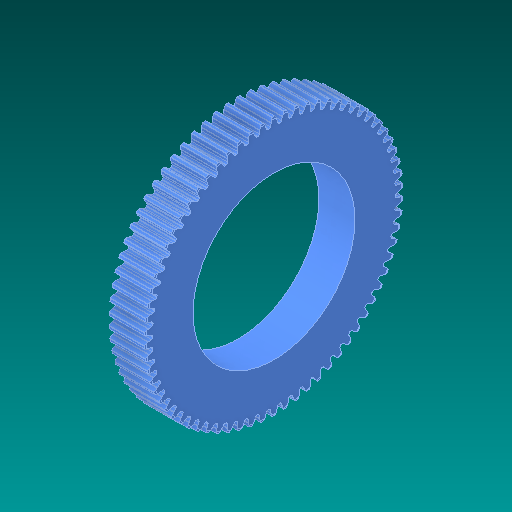
# Autodesk Inventor part: GEYK1.0-70-10-B-10K.0_t
Saved by Autodesk Inventor 2020 (Build 240168000, 168)
## iProperties
Created: 2022-11-14
Part Number: GEYK1.0-70-10-B-10K.0_t
Material: Generic
Catalog Web Link: www.cadenas.de
Description: GEY_teeth-Plastic Bonded Spur Gears
Vendor: MISUMI
Document SubType Name: Modeling
Designer: psAdmin
Manufacturer: MISUMI
Mass: 22.3714 g
Surface Area: 101.789 cm^2
Volume: 22.3714 cm^3
Density: 1 g/cm^3
Appearance: PSOLRGB-87-140-238
Category: PARTsolutions
Company: MISUMI
PSOL_IDENT_0: {$CADENAS_DATA/23d-libs/misumi/metric/54_spur_gears/gey_teeth.prj},214 {VTYP=3D},{NB=GEYK1.0-70-10-B
PSOL_IDENT_1: -10K.0_t},{LINA=GEYK1.0-70-10-B-10K.0},{NN=GEY_teeth},{DATE=07.06.2021 01:25:59},{GEOMDATE=22.08.201
PSOL_IDENT_2: 6 07:24:18},{VERSION=},{LINEID=10},{WBVAR=SHS,NT,PS,ALT1,ALT2,BS},{WBNUMERIC=NT,BS}  {NB=GEYK1.0-70-
PSOL_IDENT_3: 10-B-10K.0_t},{LINA=GEYK1.0-70-10-B-10K.0},{KT=DUMMY},{PN=GEYK1.0-70-10-B-10K.0},{SHS=K},{SHSPN=K},{
PSOL_IDENT_4: GEAKBH=0},{MAT=MC Nylon},{MATC=S25C},{AC=Set Screw},{MOD=1.0},{NT=70},{NTA=30,32,34,35,36,38,40,42,4
PSOL_IDENT_5: 5,48,50,52,56,60,70,75},{B=10},{TS=B},{TSA='B','B'},{PS=10K},{PSA= '10N','10N','10K','10K','11N','11
PSOL_IDENT_6: N','12N','12N','13N','13N','14N','14N','15N','15N','16N','16N','17N','17N','18N','18N','19N','19N','
PSOL_IDENT_7: 20N','20N','21N','21N','22N','22N','23N','23N','24N','24N'},{PS1= '10','10','11','11','12','12','13'
PSOL_IDENT_8: ,'13','14','14','15','15','16','16','17','17','18','18','19','19','20','20','21','21','22','22','23'
PSOL_IDENT_9: ,'23','24','24','25','25','26','26','27','27','28','28'},{PS2= '10N','10N','10K','10K','11N','11N','
PSOL_IDENT_10: 12N','12N','13N','13N','14N','14N','15N','15N','16N','16N','17N','17N','18N','18N','19N','19N','20N'
PSOL_IDENT_11: ,'20N','21N','21N','22N','22N','23N','23N','24N','24N'},{P=10.00},{DD=70.0},{D=72.0},{G=67.5},{H=40}
PSOL_IDENT_12: ,{E=45},{L=20},{LL1=10},{LL2=5.000},{M=M4},{M2=4},{ACSS=M4x3},{TT=0},{BB=4},{ALT1=},{ALTA='','w/o Se
PSOL_IDENT_13: t Screw', '-KC90', 'with KC90 (Set Screw)', '-KC120', 'with KC120 (Set Screw)'},{SCREWL=3},{PLANE=20
PSOL_IDENT_14: },{PLANE1=20},{ALT2=},{ALT2A='','w/o Boss Cut','-BS','with BS (Boss Cut)'},{BS=0.0},{BSA=0},{BSMIN=7
PSOL_IDENT_15: .0},{BSMAX=9.5},{MOD3D=1},{D1=1.285714},{D2=2.571429},{D3=20},{D4=0.1},{D5=11.666667},{D6=10.769231}
PSOL_IDENT_16: ,{D7=0.85},{D8=0.5},{D9=0.82917},{S1=15},{S2=0.5}
NB: GEYK1.0-70-10-B-10K.0_t
NN: GEY_teeth
NT: 70
NBSYN: $PN._t
LINA: GEYK1.0-70-10-B-10K.0
CATALOG: Misumi
SHS: Key Groove Hole+Tap
MAT: MC Nylon
MATC: S25C
MOD: 1.0
B: 10
PS: 10K
L: 20
LL1: 10
ALT1: w/o Set Screw
ALT2: w/o Boss Cut
BS: 0
SUPPLIER: MISUMI
ARTICLENO: GEYK1.0-70-10-B-10K.0_t
BOMINFO: GEYK1.0-70-10-B-10K.0
CREATOR: CADENAS GmbH
d3: 0.000 mm
Title: GEYK1.0-70-10-B-10K.0
Author: Cadenas PARTsolutions
Comments: Plastic Bonded Spur Gears
Autodesk Inventor part; units mm, degrees
(part 1 of 2)
sketch "_____2" plane through (0, 0, 0) normal (0, 0, 1) x (1, 0, 0)
  line L0 (0, 0) -> (-10, 0)
  line L1 (-10, 22.5) -> (0, 22.5)
  line L2 (0, 22.5) -> (0, 35.5)
  line L3 (0, 35.5) -> (-0.6699, 38)
  line L4 (-0.6699, 38) -> (-9.3301, 38)
  line L5 (-9.3301, 38) -> (-10, 35.5)
  line L6 (-10, 35.5) -> (-10, 22.5)
  constraints: 14 end point
revolve "Revolution1" add sketch "_____2" angle 360 about axis through (0, 0, 0) along (1, 0, 0)
sketch "Sketch_2" plane through (0, 0, 0) normal (1, 0, 0) x (0, 1, 0)
  circle A0 centre (0, 0) radius 144
  arc A1 (1.2884, 35.9769) -> (1.1952, 35.9213) centre (1.2849, 35.877) ccw
  arc A2 (1.1952, 35.9213) -> (0.7853, 34.9912) centre (11.6561, 30.756) ccw
  arc A3 (0.7853, 34.9912) -> (0.7497, 34.8755) centre (1.5579, 34.6902) ccw
  arc A4 (0.5416, 34.1021) -> (0.7497, 34.8755) centre (-9.7463, 37.2859) ccw
  arc A5 (0.063, 33.7499) -> (0.5416, 34.1021) centre (0.0639, 34.2499) ccw
  arc A6 (0.063, 33.7499) -> (-0.063, 33.7499) centre (0, 0) ccw
  arc A7 (-0.5416, 34.1021) -> (-0.063, 33.7499) centre (-0.0639, 34.2499) ccw
  arc A8 (-0.7497, 34.8755) -> (-0.5416, 34.1021) centre (9.7463, 37.2859) ccw
  arc A9 (-0.7497, 34.8755) -> (-0.7853, 34.9912) centre (-1.5579, 34.6902) ccw
  arc A10 (-0.7853, 34.9912) -> (-1.1952, 35.9213) centre (-11.6561, 30.756) ccw
  arc A11 (-1.1952, 35.9213) -> (-1.2884, 35.9769) centre (-1.2849, 35.877) ccw
  arc A12 (-1.2884, 35.9769) -> (-1.9417, 35.9476) centre (0, 0) ccw
  arc A13 (-1.9417, 35.9476) -> (-2.0296, 35.8838) centre (-1.9363, 35.8477) ccw
  arc A14 (-2.0296, 35.8838) -> (-2.3544, 34.9207) centre (8.8523, 31.677) ccw
  arc A15 (-2.3544, 34.9207) -> (-2.3795, 34.8023) centre (-1.5579, 34.6902) ccw
  arc A16 (-2.5175, 34.0134) -> (-2.3795, 34.8023) centre (-13.0493, 36.2622) ccw
  arc A17 (-2.9626, 33.6197) -> (-2.5175, 34.0134) centre (-3.0065, 34.1178) ccw
  arc A18 (-2.9626, 33.6197) -> (-3.0881, 33.6084) centre (0, 0) ccw
  arc A19 (-3.5963, 33.9163) -> (-3.0881, 33.6084) centre (-3.1338, 34.1063) ccw
  arc A20 (-3.8729, 34.6679) -> (-3.5963, 33.9163) centre (6.3647, 38.0095) ccw
  arc A21 (-3.8729, 34.6679) -> (-3.9188, 34.7799) centre (-4.6613, 34.4109) ccw
  arc A22 (-3.9188, 34.7799) -> (-4.4104, 35.6695) centre (-14.3661, 29.5873) ccw
  arc A23 (-4.4104, 35.6695) -> (-4.5082, 35.7166) centre (-4.4957, 35.6174) ccw
  arc A24 (-4.5082, 35.7166) -> (-5.1562, 35.6288) centre (0, 0) ccw
  arc A25 (-5.1562, 35.6288) -> (-5.238, 35.5574) centre (-5.1419, 35.5299) ccw
  arc A26 (-5.238, 35.5574) -> (-5.4752, 34.5691) centre (5.9771, 32.343) ccw
  arc A27 (-5.4752, 34.5691) -> (-5.4896, 34.4489) centre (-4.6613, 34.4109) ccw
  arc A28 (-5.5563, 33.6508) -> (-5.4896, 34.4489) centre (-16.2473, 34.9465) ccw
  arc A29 (-5.9643, 33.2188) -> (-5.5563, 33.6508) centre (-6.0527, 33.7109) ccw
  arc A30 (-5.9643, 33.2188) -> (-6.0883, 33.1963) centre (0, 0) ccw
  arc A31 (-6.622, 33.4574) -> (-6.0883, 33.1963) centre (-6.1785, 33.6881) ccw
  arc A32 (-6.965, 34.1812) -> (-6.622, 33.4574) centre (2.932, 38.427) ccw
  arc A33 (-6.965, 34.1812) -> (-7.0206, 34.2886) centre (-7.7271, 33.8545) ccw
  arc A34 (-7.0206, 34.2886) -> (-7.59, 35.1306) centre (-16.9605, 28.1804) ccw
  arc A35 (-7.59, 35.1306) -> (-7.6917, 35.1687) centre (-7.6703, 35.071) ccw
  arc A36 (-7.6917, 35.1687) -> (-8.3292, 35.0232) centre (0, 0) ccw
  arc A37 (-8.3292, 35.0232) -> (-8.4042, 34.9447) centre (-8.306, 34.9259) ccw
  arc A38 (-8.4042, 34.9447) -> (-8.5519, 33.9391) centre (3.0538, 32.7486) ccw
  arc A39 (-8.5519, 33.9391) -> (-8.5554, 33.8182) centre (-7.7271, 33.8545) ccw
  arc A40 (-8.5504, 33.0173) -> (-8.5554, 33.8182) centre (-19.3145, 33.3494) ccw
  arc A41 (-8.918, 32.5504) -> (-8.5504, 33.0173) centre (-9.0501, 33.0327) ccw
  arc A42 (-8.918, 32.5504) -> (-9.0395, 32.5169) centre (0, 0) ccw
  arc A43 (-9.5945, 32.7291) -> (-9.0395, 32.5169) centre (-9.1734, 32.9987) ccw
  arc A44 (-10.0009, 33.4192) -> (-9.5945, 32.7291) centre (-0.5244, 38.5351) ccw
  arc A45 (-10.0009, 33.4192) -> (-10.066, 33.5213) centre (-10.7307, 33.0256) ccw
  arc A46 (-10.066, 33.5213) -> (-10.7085, 34.3088) centre (-19.4183, 26.5467) ccw
  arc A47 (-10.7085, 34.3088) -> (-10.8132, 34.3377) centre (-10.7832, 34.2423) ccw
  arc A48 (-10.8132, 34.3377) -> (-11.4351, 34.1356) centre (0, 0) ccw
  arc A49 (-11.4351, 34.1356) -> (-11.5028, 34.0507) centre (-11.4033, 34.0408) ccw
  arc A50 (-11.5028, 34.0507) -> (-11.5598, 33.0359) centre (0.106, 32.8905) ccw
  arc A51 (-11.5598, 33.0359) -> (-11.5524, 32.9151) centre (-10.7307, 33.0256) ccw
  arc A52 (-11.4756, 32.1179) -> (-11.5524, 32.9151) centre (-22.2261, 31.4838) ccw
  arc A53 (-11.7999, 31.62) -> (-11.4756, 32.1179) centre (-11.9747, 32.0885) ccw
  arc A54 (-11.7999, 31.62) -> (-11.9179, 31.5757) centre (0, 0) ccw
  arc A55 (-12.4897, 31.7373) -> (-11.9179, 31.5757) centre (-12.0944, 32.0435) ccw
  arc A56 (-12.9563, 32.3882) -> (-12.4897, 31.7373) centre (-3.9765, 38.333) ccw
  arc A57 (-12.9563, 32.3882) -> (-13.0303, 32.484) centre (-13.6479, 31.9307) ccw
  arc A58 (-13.0303, 32.484) -> (-13.7408, 33.2108) centre (-21.7197, 24.6991) ccw
  arc A59 (-13.7408, 33.2108) -> (-13.8477, 33.2301) centre (-13.8092, 33.1378) ccw
  arc A60 (-13.8477, 33.2301) -> (-14.449, 32.9731) centre (0, 0) ccw
  arc A61 (-14.449, 32.9731) -> (-14.5088, 32.8825) centre (-14.4088, 32.8815) ccw
  arc A62 (-14.5088, 32.8825) -> (-14.4745, 31.8667) centre (-2.8427, 32.7676) ccw
  arc A63 (-14.4745, 31.8667) -> (-14.4564, 31.747) centre (-13.6479, 31.9307) ccw
  arc A64 (-14.3084, 30.9599) -> (-14.4564, 31.747) centre (-24.9588, 29.3647) ccw
  arc A65 (-14.5868, 30.435) -> (-14.3084, 30.9599) centre (-14.8029, 30.8859) ccw
  arc A66 (-14.5868, 30.435) -> (-14.7003, 30.3803) centre (0, 0) ccw
  arc A67 (-15.2843, 30.49) -> (-14.7003, 30.3803) centre (-14.9181, 30.8304) ccw
  arc A68 (-15.8074, 31.0964) -> (-15.2843, 30.49) centre (-7.3967, 37.8222) ccw
  arc A69 (-15.8074, 31.0964) -> (-15.8897, 31.1852) centre (-16.4552, 30.5788) ccw
  arc A70 (-15.8897, 31.1852) -> (-16.6625, 31.8454) centre (-23.8463, 22.6528) ccw
  arc A71 (-16.6625, 31.8454) -> (-16.7707, 31.8551) centre (-16.7241, 31.7666) ccw
  arc A72 (-16.7707, 31.8551) -> (-17.3465, 31.5452) centre (0, 0) ccw
  arc A73 (-17.3465, 31.5452) -> (-17.398, 31.4496) centre (-17.2983, 31.4576) ccw
  arc A74 (-17.398, 31.4496) -> (-17.2728, 30.4409) centre (-5.7685, 32.3808) ccw
  arc A75 (-17.2728, 30.4409) -> (-17.244, 30.3234) centre (-16.4552, 30.5788) ccw
  arc A76 (-17.026, 29.5527) -> (-17.244, 30.3234) centre (-27.4906, 27.0092) ccw
  arc A77 (-17.2562, 29.0049) -> (-17.026, 29.5527) centre (-17.5119, 29.4346) ccw
  arc A78 (-17.2562, 29.0049) -> (-17.3644, 28.9403) centre (0, 0) ccw
  arc A79 (-17.9559, 28.9971) -> (-17.3644, 28.9403) centre (-17.6216, 29.369) ccw
  arc A80 (-18.5312, 29.5543) -> (-17.9559, 28.9971) centre (-10.7572, 37.0069) ccw
  arc A81 (-18.5312, 29.5543) -> (-18.6211, 29.6353) centre (-19.13, 28.9807) ccw
  arc A82 (-18.6211, 29.6353) -> (-19.45, 30.2236) centre (-25.7809, 20.424) ccw
  arc A83 (-19.45, 30.2236) -> (-19.5586, 30.2235) centre (-19.5043, 30.1396) ccw
  arc A84 (-19.5586, 30.2235) -> (-20.1043, 29.8633) centre (0, 0) ccw
  arc A85 (-20.1043, 29.8633) -> (-20.1471, 29.7634) centre (-20.0485, 29.7803) ccw
  arc A86 (-20.1471, 29.7634) -> (-19.932, 28.7701) centre (-8.6479, 31.7334) ccw
  arc A87 (-19.932, 28.7701) -> (-19.8928, 28.6556) centre (-19.13, 28.9807) ccw
  arc A88 (-19.6066, 27.9075) -> (-19.8928, 28.6556) centre (-29.801, 24.4362) ccw
  arc A89 (-19.7868, 27.3413) -> (-19.6066, 27.9075) centre (-20.0799, 27.7464) ccw
  arc A90 (-19.7868, 27.3413) -> (-19.8887, 27.2672) centre (0, 0) ccw
  arc A91 (-20.4829, 27.2709) -> (-19.8887, 27.2672) centre (-20.1833, 27.6712) ccw
  arc A92 (-21.1059, 27.7742) -> (-20.4829, 27.2709) centre (-14.0312, 35.8937) ccw
  arc A93 (-21.1059, 27.7742) -> (-21.2027, 27.8469) centre (-21.6508, 27.1492) ccw
  arc A94 (-21.2027, 27.8469) -> (-22.0809, 28.3584) centre (-27.5079, 18.0308) ccw
  arc A95 (-22.0809, 28.3584) -> (-22.1891, 28.3486) centre (-22.1275, 28.2699) ccw
  arc A96 (-22.1891, 28.3486) -> (-22.7003, 27.9409) centre (0, 0) ccw
  arc A97 (-22.7003, 27.9409) -> (-22.7339, 27.8377) centre (-22.6373, 27.8633) ccw
  arc A98 (-22.7339, 27.8377) -> (-22.4306, 26.8676) centre (-11.4577, 30.8305) ccw
  arc A99 (-22.4306, 26.8676) -> (-22.3813, 26.757) centre (-21.6508, 27.1492) ccw
  arc A100 (-22.0293, 26.0377) -> (-22.3813, 26.757) centre (-31.8715, 21.6665) ccw
  arc A101 (-22.158, 25.4576) -> (-22.0293, 26.0377) centre (-22.4862, 25.8347) ccw
  arc A102 (-22.158, 25.4576) -> (-22.2528, 25.3747) centre (0, 0) ccw
  arc A103 (-22.845, 25.325) -> (-22.2528, 25.3747) centre (-22.5825, 25.7506) ccw
  arc A104 (-23.5106, 25.7705) -> (-22.845, 25.325) centre (-17.1922, 34.4914) ccw
  arc A105 (-23.5106, 25.7705) -> (-23.6135, 25.8342) centre (-23.9973, 25.0992) ccw
  arc A106 (-23.6135, 25.8342) -> (-24.5341, 26.2649) centre (-29.0134, 15.4924) ccw
  arc A107 (-24.5341, 26.2649) -> (-24.6409, 26.2455) centre (-24.5725, 26.1726) ccw
  arc A108 (-24.6409, 26.2455) -> (-25.1135, 25.7936) centre (0, 0) ccw
  arc A109 (-25.1135, 25.7936) -> (-25.1378, 25.6877) centre (-25.0438, 25.722) ccw
  arc A110 (-25.1378, 25.6877) -> (-24.7487, 24.7487) centre (-14.1751, 29.6793) ccw
  arc A111 (-24.7487, 24.7487) -> (-24.6897, 24.6431) centre (-23.9973, 25.0992) ccw
  arc A112 (-24.2746, 23.9582) -> (-24.6897, 24.6431) centre (-33.6854, 18.7224) ccw
  arc A113 (-24.3508, 23.3689) -> (-24.2746, 23.9582) centre (-24.7115, 23.7151) ccw
  arc A114 (-24.3508, 23.3689) -> (-24.4378, 23.2778) centre (0, 0) ccw
  arc A115 (-25.0231, 23.1753) -> (-24.4378, 23.2778) centre (-24.7999, 23.6226) ccw
  arc A116 (-25.726, 23.5592) -> (-25.0231, 23.1753) centre (-20.2148, 32.8115) ccw
  arc A117 (-25.726, 23.5592) -> (-25.8342, 23.6135) centre (-26.1505, 22.847) ccw
  arc A118 (-25.8342, 23.6135) -> (-26.7897, 23.96) centre (-30.2854, 12.8293) ccw
  arc A119 (-26.7897, 23.96) -> (-26.8943, 23.931) centre (-26.8196, 23.8646) ccw
  arc A120 (-26.8943, 23.931) -> (-27.3246, 23.4386) centre (0, 0) ccw
  arc A121 (-27.3246, 23.4386) -> (-27.3392, 23.331) centre (-27.2487, 23.3735) ccw
  arc A122 (-27.3392, 23.331) -> (-26.8676, 22.4306) centre (-16.7785, 28.2892) ccw
  arc A123 (-26.8676, 22.4306) -> (-26.7993, 22.3307) centre (-26.1505, 22.847) ccw
  arc A124 (-26.3244, 21.6857) -> (-26.7993, 22.3307) centre (-35.228, 15.6275) ccw
  arc A125 (-26.3475, 21.092) -> (-26.3244, 21.6857) centre (-26.7378, 21.4045) ccw
  arc A126 (-26.3475, 21.092) -> (-26.426, 20.9935) centre (0, 0) ccw
  arc A127 (-26.9998, 20.8389) -> (-26.426, 20.9935) centre (-26.8175, 21.3045) ccw
  arc A128 (-27.7342, 21.1584) -> (-26.9998, 20.8389) centre (-23.0746, 30.8673) ccw
  arc A129 (-27.7342, 21.1584) -> (-27.8469, 21.2027) centre (-28.0932, 20.4109) ccw
  arc A130 (-27.8469, 21.2027) -> (-28.8296, 21.4621) centre (-31.3135, 10.0629) ccw
  arc A131 (-28.8296, 21.4621) -> (-28.9312, 21.4239) centre (-28.8509, 21.3644) ccw
  arc A132 (-28.9312, 21.4239) -> (-29.3156, 20.8949) centre (0, 0) ccw
  arc A133 (-29.3156, 20.8949) -> (-29.3205, 20.7864) centre (-29.2342, 20.8368) ccw
  arc A134 (-29.3205, 20.7864) -> (-28.7701, 19.932) centre (-19.2468, 26.6713) ccw
  arc A135 (-28.7701, 19.932) -> (-28.6931, 19.8385) centre (-28.0932, 20.4109) ccw
  arc A136 (-28.1624, 19.2387) -> (-28.6931, 19.8385) centre (-36.487, 12.4067) ccw
  arc A137 (-28.1321, 18.6453) -> (-28.1624, 19.2387) centre (-28.5489, 18.9215) ccw
  arc A138 (-28.1321, 18.6453) -> (-28.2015, 18.5402) centre (0, 0) ccw
  arc A139 (-28.7591, 18.3348) -> (-28.2015, 18.5402) centre (-28.6193, 18.8148) ccw
  arc A140 (-29.5192, 18.5871) -> (-28.7591, 18.3348) centre (-25.7486, 28.6747) ccw
  arc A141 (-29.5192, 18.5871) -> (-29.6353, 18.6211) centre (-29.8098, 17.8105) ccw
  arc A142 (-29.6353, 18.6211) -> (-30.6374, 18.7914) centre (-32.0894, 7.2155) ccw
  arc A143 (-30.6374, 18.7914) -> (-30.7352, 18.7443) centre (-30.6498, 18.6922) ccw
  arc A144 (-30.7352, 18.7443) -> (-31.0706, 18.1829) centre (0, 0) ccw
  arc A145 (-31.0706, 18.1829) -> (-31.0657, 18.0745) centre (-30.9843, 18.1324) ccw
  arc A146 (-31.0657, 18.0745) -> (-30.4409, 17.2728) centre (-21.5601, 24.8386) ccw
  arc A147 (-30.4409, 17.2728) -> (-30.3559, 17.1866) centre (-29.8098, 17.8105) ccw
  arc A148 (-29.7735, 16.6368) -> (-30.3559, 17.1866) centre (-37.4523, 9.0861) ccw
  arc A149 (-29.6902, 16.0485) -> (-29.7735, 16.6368) centre (-30.1301, 16.2863) ccw
  arc A150 (-29.6902, 16.0485) -> (-29.7499, 15.9376) centre (0, 0) ccw
  arc A151 (-30.2868, 15.683) -> (-29.7499, 15.9376) centre (-30.1906, 16.1737) ccw
  arc A152 (-31.0665, 15.8662) -> (-30.2868, 15.683) centre (-28.2154, 26.2511) ccw
  arc A153 (-31.0665, 15.8662) -> (-31.1852, 15.8897) centre (-31.2863, 15.0667) ccw
  arc A154 (-31.1852, 15.8897) -> (-32.1985, 15.9695) centre (-32.607, 4.31) ccw
  arc A155 (-32.1985, 15.9695) -> (-32.2917, 15.9137) centre (-32.202, 15.8695) ccw
  arc A156 (-32.2917, 15.9137) -> (-32.5754, 15.3246) centre (0, 0) ccw
  arc A157 (-32.5754, 15.3246) -> (-32.5609, 15.217) centre (-32.4849, 15.282) ccw
  arc A158 (-32.5609, 15.217) -> (-31.8667, 14.4745) centre (-23.6998, 22.806) ccw
  arc A159 (-31.8667, 14.4745) -> (-31.7743, 14.3964) centre (-31.2863, 15.0667) ccw
  arc A160 (-31.145, 13.901) -> (-31.7743, 14.3964) centre (-38.116, 5.6923) ccw
  arc A161 (-31.0092, 13.3225) -> (-31.145, 13.901) centre (-31.4686, 13.5199) ccw
  arc A162 (-31.0092, 13.3225) -> (-31.0588, 13.2066) centre (0, 0) ccw
  arc A163 (-31.5707, 12.905) -> (-31.0588, 13.2066) centre (-31.5189, 13.4023) ccw
  arc A164 (-32.3637, 13.0175) -> (-31.5707, 12.905) centre (-30.4549, 23.6163) ccw
  arc A165 (-32.3637, 13.0175) -> (-32.484, 13.0303) centre (-32.5109, 12.2015) ccw
  arc A166 (-32.484, 13.0303) -> (-33.5004, 13.0189) centre (-32.8621, 1.3697) ccw
  arc A167 (-33.5004, 13.0189) -> (-33.5882, 12.9551) centre (-33.4949, 12.9191) ccw
  arc A168 (-33.5882, 12.9551) -> (-33.8179, 12.3429) centre (0, 0) ccw
  arc A169 (-33.8179, 12.3429) -> (-33.7938, 12.237) centre (-33.724, 12.3086) ccw
  arc A170 (-33.7938, 12.237) -> (-33.0359, 11.5598) centre (-25.6487, 20.5897) ccw
  arc A171 (-33.0359, 11.5598) -> (-32.9369, 11.4902) centre (-32.5109, 12.2015) ccw
  arc A172 (-32.2657, 11.0532) -> (-32.9369, 11.4902) centre (-38.4728, 2.2527) ccw
  arc A173 (-32.0786, 10.4892) -> (-32.2657, 11.0532) centre (-32.5539, 10.6446) ccw
  arc A174 (-32.0786, 10.4892) -> (-32.1176, 10.3694) centre (0, 0) ccw
  arc A175 (-32.6004, 10.0231) -> (-32.1176, 10.3694) centre (-32.5934, 10.523) ccw
  arc A176 (-33.4003, 10.0641) -> (-32.6004, 10.0231) centre (-32.4493, 20.7912) ccw
  arc A177 (-33.4003, 10.0641) -> (-33.5213, 10.066) centre (-33.4738, 9.2382) ccw
  arc A178 (-33.5213, 10.066) -> (-34.5325, 9.9636) centre (-32.8526, -1.5815) ccw
  arc A179 (-34.5325, 9.9636) -> (-34.6143, 9.8921) centre (-34.5181, 9.8646) ccw
  arc A180 (-34.6143, 9.8921) -> (-34.7882, 9.2618) centre (0, 0) ccw
  arc A181 (-34.7882, 9.2618) -> (-34.7547, 9.1585) centre (-34.6916, 9.236) ccw
  arc A182 (-34.7547, 9.1585) -> (-33.9391, 8.5519) centre (-27.3911, 18.2077) ccw
  arc A183 (-33.9391, 8.5519) -> (-33.8343, 8.4915) centre (-33.4738, 9.2382) ccw
  arc A184 (-33.1266, 8.1164) -> (-33.8343, 8.4915) centre (-38.5198, -1.205) ccw
  arc A185 (-32.8897, 7.5715) -> (-33.1266, 8.1164) centre (-33.377, 7.6837) ccw
  arc A186 (-32.8897, 7.5715) -> (-32.9178, 7.4487) centre (0, 0) ccw
  arc A187 (-33.3676, 7.0604) -> (-32.9178, 7.4487) centre (-33.4054, 7.559) ccw
  arc A188 (-34.1679, 7.0296) -> (-33.3676, 7.0604) centre (-34.1823, 17.7988) ccw
  arc A189 (-34.1679, 7.0296) -> (-34.2886, 7.0206) centre (-34.1671, 6.2004) ccw
  arc A190 (-34.2886, 7.0206) -> (-35.2866, 6.828) centre (-32.5786, -4.52) ccw
  arc A191 (-35.2866, 6.828) -> (-35.3616, 6.7495) centre (-35.2634, 6.7307) ccw
  arc A192 (-35.3616, 6.7495) -> (-35.4784, 6.1061) centre (0, 0) ccw
  arc A193 (-35.4784, 6.1061) -> (-35.4357, 6.0062) centre (-35.3798, 6.0891) ccw
  arc A194 (-35.4357, 6.0062) -> (-34.5691, 5.4752) centre (-28.913, 15.6791) ccw
  arc A195 (-34.5691, 5.4752) -> (-34.4592, 5.4244) centre (-34.1671, 6.2004) ccw
  arc A196 (-33.7208, 5.1143) -> (-34.4592, 5.4244) centre (-38.2567, -4.6531) ccw
  arc A197 (-33.436, 4.5928) -> (-33.7208, 5.1143) centre (-33.9314, 4.6608) ccw
  arc A198 (-33.436, 4.5928) -> (-33.453, 4.4679) centre (0, 0) ccw
  arc A199 (-33.8662, 4.041) -> (-33.453, 4.4679) centre (-33.9486, 4.5341) ccw
  arc A200 (-34.6605, 3.9385) -> (-33.8662, 4.041) centre (-35.6402, 14.6631) ccw
  arc A201 (-34.6605, 3.9385) -> (-34.7799, 3.9188) centre (-34.5854, 3.1127) ccw
  arc A202 (-34.7799, 3.9188) -> (-35.7566, 3.6374) centre (-32.0423, -7.4222) ccw
  arc A203 (-35.7566, 3.6374) -> (-35.8243, 3.5525) centre (-35.7248, 3.5426) ccw
  arc A204 (-35.8243, 3.5525) -> (-35.8829, 2.9013) centre (0, 0) ccw
  arc A205 (-35.8829, 2.9013) -> (-35.8315, 2.8056) centre (-35.7832, 2.8932) ccw
  arc A206 (-35.8315, 2.8056) -> (-34.9207, 2.3544) centre (-30.202, 13.0242) ccw
  arc A207 (-34.9207, 2.3544) -> (-34.8068, 2.3137) centre (-34.5854, 3.1127) ccw
  arc A208 (-34.0435, 2.071) -> (-34.8068, 2.3137) centre (-37.6856, -8.0636) ccw
  arc A209 (-33.7131, 1.5771) -> (-34.0435, 2.071) centre (-34.2126, 1.6005) ccw
  arc A210 (-33.7131, 1.5771) -> (-33.7188, 1.4513) centre (0, 0) ccw
  arc A211 (-34.0921, 0.989) -> (-33.7188, 1.4513) centre (-34.2183, 1.4728) ccw
  arc A212 (-34.874, 0.8157) -> (-34.0921, 0.989) centre (-36.8111, 11.4093) ccw
  arc A213 (-34.874, 0.8157) -> (-34.9912, 0.7853) centre (-34.7251, 0) ccw
  arc A214 (-34.9912, 0.7853) -> (-35.9387, 0.4176) centre (-31.2479, -10.2645) ccw
  arc A215 (-35.9387, 0.4176) -> (-35.9985, 0.3269) centre (-35.8985, 0.326) ccw
  arc A216 (-35.9985, 0.3269) -> (-35.9985, -0.3269) centre (0, 0) ccw
  arc A217 (-35.9985, -0.3269) -> (-35.9387, -0.4176) centre (-35.8985, -0.326) ccw
  arc A218 (-35.9387, -0.4176) -> (-34.9912, -0.7853) centre (-31.2479, 10.2645) ccw
  arc A219 (-34.9912, -0.7853) -> (-34.874, -0.8157) centre (-34.7251, 0) ccw
  arc A220 (-34.0921, -0.989) -> (-34.874, -0.8157) centre (-36.8111, -11.4093) ccw
  arc A221 (-33.7188, -1.4513) -> (-34.0921, -0.989) centre (-34.2183, -1.4728) ccw
  arc A222 (-33.7188, -1.4513) -> (-33.7131, -1.5771) centre (0, 0) ccw
  arc A223 (-34.0435, -2.071) -> (-33.7131, -1.5771) centre (-34.2126, -1.6005) ccw
  arc A224 (-34.8068, -2.3137) -> (-34.0435, -2.071) centre (-37.6856, 8.0636) ccw
  arc A225 (-34.8068, -2.3137) -> (-34.9207, -2.3544) centre (-34.5854, -3.1127) ccw
  arc A226 (-34.9207, -2.3544) -> (-35.8315, -2.8056) centre (-30.202, -13.0242) ccw
  arc A227 (-35.8315, -2.8056) -> (-35.8829, -2.9013) centre (-35.7832, -2.8932) ccw
  arc A228 (-35.8829, -2.9013) -> (-35.8243, -3.5525) centre (0, 0) ccw
  arc A229 (-35.8243, -3.5525) -> (-35.7566, -3.6374) centre (-35.7248, -3.5426) ccw
  arc A230 (-35.7566, -3.6374) -> (-34.7799, -3.9188) centre (-32.0423, 7.4222) ccw
  arc A231 (-34.7799, -3.9188) -> (-34.6605, -3.9385) centre (-34.5854, -3.1127) ccw
  arc A232 (-33.8662, -4.041) -> (-34.6605, -3.9385) centre (-35.6402, -14.6631) ccw
  arc A233 (-33.453, -4.4679) -> (-33.8662, -4.041) centre (-33.9486, -4.5341) ccw
  arc A234 (-33.453, -4.4679) -> (-33.436, -4.5928) centre (0, 0) ccw
  arc A235 (-33.7208, -5.1143) -> (-33.436, -4.5928) centre (-33.9314, -4.6608) ccw
  arc A236 (-34.4592, -5.4244) -> (-33.7208, -5.1143) centre (-38.2567, 4.6531) ccw
  arc A237 (-34.4592, -5.4244) -> (-34.5691, -5.4752) centre (-34.1671, -6.2004) ccw
  arc A238 (-34.5691, -5.4752) -> (-35.4357, -6.0062) centre (-28.913, -15.6791) ccw
  arc A239 (-35.4357, -6.0062) -> (-35.4784, -6.1061) centre (-35.3798, -6.0891) ccw
  arc A240 (-35.4784, -6.1061) -> (-35.3616, -6.7495) centre (0, 0) ccw
  arc A241 (-35.3616, -6.7495) -> (-35.2866, -6.828) centre (-35.2634, -6.7307) ccw
  arc A242 (-35.2866, -6.828) -> (-34.2886, -7.0206) centre (-32.5786, 4.52) ccw
  arc A243 (-34.2886, -7.0206) -> (-34.1679, -7.0296) centre (-34.1671, -6.2004) ccw
  arc A244 (-33.3676, -7.0604) -> (-34.1679, -7.0296) centre (-34.1823, -17.7988) ccw
  arc A245 (-32.9178, -7.4487) -> (-33.3676, -7.0604) centre (-33.4054, -7.559) ccw
  arc A246 (-32.9178, -7.4487) -> (-32.8897, -7.5715) centre (0, 0) ccw
  arc A247 (-33.1266, -8.1164) -> (-32.8897, -7.5715) centre (-33.377, -7.6837) ccw
  arc A248 (-33.8343, -8.4915) -> (-33.1266, -8.1164) centre (-38.5198, 1.205) ccw
  arc A249 (-33.8343, -8.4915) -> (-33.9391, -8.5519) centre (-33.4738, -9.2382) ccw
  arc A250 (-33.9391, -8.5519) -> (-34.7547, -9.1585) centre (-27.3911, -18.2077) ccw
  arc A251 (-34.7547, -9.1585) -> (-34.7882, -9.2618) centre (-34.6916, -9.236) ccw
  arc A252 (-34.7882, -9.2618) -> (-34.6143, -9.8921) centre (0, 0) ccw
  arc A253 (-34.6143, -9.8921) -> (-34.5325, -9.9636) centre (-34.5181, -9.8646) ccw
  arc A254 (-34.5325, -9.9636) -> (-33.5213, -10.066) centre (-32.8526, 1.5815) ccw
  arc A255 (-33.5213, -10.066) -> (-33.4003, -10.0641) centre (-33.4738, -9.2382) ccw
  arc A256 (-32.6004, -10.0231) -> (-33.4003, -10.0641) centre (-32.4493, -20.7912) ccw
  arc A257 (-32.1176, -10.3694) -> (-32.6004, -10.0231) centre (-32.5934, -10.523) ccw
  arc A258 (-32.1176, -10.3694) -> (-32.0786, -10.4892) centre (0, 0) ccw
  arc A259 (-32.2657, -11.0532) -> (-32.0786, -10.4892) centre (-32.5539, -10.6446) ccw
  arc A260 (-32.9369, -11.4902) -> (-32.2657, -11.0532) centre (-38.4728, -2.2527) ccw
  arc A261 (-32.9369, -11.4902) -> (-33.0359, -11.5598) centre (-32.5109, -12.2015) ccw
  arc A262 (-33.0359, -11.5598) -> (-33.7938, -12.237) centre (-25.6487, -20.5897) ccw
  arc A263 (-33.7938, -12.237) -> (-33.8179, -12.3429) centre (-33.724, -12.3086) ccw
  arc A264 (-33.8179, -12.3429) -> (-33.5882, -12.9551) centre (0, 0) ccw
  arc A265 (-33.5882, -12.9551) -> (-33.5004, -13.0189) centre (-33.4949, -12.9191) ccw
  arc A266 (-33.5004, -13.0189) -> (-32.484, -13.0303) centre (-32.8621, -1.3697) ccw
  arc A267 (-32.484, -13.0303) -> (-32.3637, -13.0175) centre (-32.5109, -12.2015) ccw
  arc A268 (-31.5707, -12.905) -> (-32.3637, -13.0175) centre (-30.4549, -23.6163) ccw
  arc A269 (-31.0588, -13.2066) -> (-31.5707, -12.905) centre (-31.5189, -13.4023) ccw
  arc A270 (-31.0588, -13.2066) -> (-31.0092, -13.3225) centre (0, 0) ccw
  arc A271 (-31.145, -13.901) -> (-31.0092, -13.3225) centre (-31.4686, -13.5199) ccw
  arc A272 (-31.7743, -14.3964) -> (-31.145, -13.901) centre (-38.116, -5.6923) ccw
  arc A273 (-31.7743, -14.3964) -> (-31.8667, -14.4745) centre (-31.2863, -15.0667) ccw
  arc A274 (-31.8667, -14.4745) -> (-32.5609, -15.217) centre (-23.6998, -22.806) ccw
  arc A275 (-32.5609, -15.217) -> (-32.5754, -15.3246) centre (-32.4849, -15.282) ccw
  arc A276 (-32.5754, -15.3246) -> (-32.2917, -15.9137) centre (0, 0) ccw
  arc A277 (-32.2917, -15.9137) -> (-32.1985, -15.9695) centre (-32.202, -15.8695) ccw
  arc A278 (-32.1985, -15.9695) -> (-31.1852, -15.8897) centre (-32.607, -4.31) ccw
  arc A279 (-31.1852, -15.8897) -> (-31.0665, -15.8662) centre (-31.2863, -15.0667) ccw
  arc A280 (-30.2868, -15.683) -> (-31.0665, -15.8662) centre (-28.2154, -26.2511) ccw
  arc A281 (-29.7499, -15.9376) -> (-30.2868, -15.683) centre (-30.1906, -16.1737) ccw
  arc A282 (-29.7499, -15.9376) -> (-29.6902, -16.0485) centre (0, 0) ccw
  arc A283 (-29.7735, -16.6368) -> (-29.6902, -16.0485) centre (-30.1301, -16.2863) ccw
  arc A284 (-30.3559, -17.1866) -> (-29.7735, -16.6368) centre (-37.4523, -9.0861) ccw
  arc A285 (-30.3559, -17.1866) -> (-30.4409, -17.2728) centre (-29.8098, -17.8105) ccw
  arc A286 (-30.4409, -17.2728) -> (-31.0657, -18.0745) centre (-21.5601, -24.8386) ccw
  arc A287 (-31.0657, -18.0745) -> (-31.0706, -18.1829) centre (-30.9843, -18.1324) ccw
  arc A288 (-31.0706, -18.1829) -> (-30.7352, -18.7443) centre (0, 0) ccw
  arc A289 (-30.7352, -18.7443) -> (-30.6374, -18.7914) centre (-30.6498, -18.6922) ccw
  arc A290 (-30.6374, -18.7914) -> (-29.6353, -18.6211) centre (-32.0894, -7.2155) ccw
  arc A291 (-29.6353, -18.6211) -> (-29.5192, -18.5871) centre (-29.8098, -17.8105) ccw
  arc A292 (-28.7591, -18.3348) -> (-29.5192, -18.5871) centre (-25.7486, -28.6747) ccw
  arc A293 (-28.2015, -18.5402) -> (-28.7591, -18.3348) centre (-28.6193, -18.8148) ccw
  arc A294 (-28.2015, -18.5402) -> (-28.1321, -18.6453) centre (0, 0) ccw
  arc A295 (-28.1624, -19.2387) -> (-28.1321, -18.6453) centre (-28.5489, -18.9215) ccw
  arc A296 (-28.6931, -19.8385) -> (-28.1624, -19.2387) centre (-36.487, -12.4067) ccw
  arc A297 (-28.6931, -19.8385) -> (-28.7701, -19.932) centre (-28.0932, -20.4109) ccw
  arc A298 (-28.7701, -19.932) -> (-29.3205, -20.7864) centre (-19.2468, -26.6713) ccw
  arc A299 (-29.3205, -20.7864) -> (-29.3156, -20.8949) centre (-29.2342, -20.8368) ccw
  arc A300 (-29.3156, -20.8949) -> (-28.9312, -21.4239) centre (0, 0) ccw
  arc A301 (-28.9312, -21.4239) -> (-28.8296, -21.4621) centre (-28.8509, -21.3644) ccw
  arc A302 (-28.8296, -21.4621) -> (-27.8469, -21.2027) centre (-31.3135, -10.0629) ccw
  arc A303 (-27.8469, -21.2027) -> (-27.7342, -21.1584) centre (-28.0932, -20.4109) ccw
  arc A304 (-26.9998, -20.8389) -> (-27.7342, -21.1584) centre (-23.0746, -30.8673) ccw
  arc A305 (-26.426, -20.9935) -> (-26.9998, -20.8389) centre (-26.8175, -21.3045) ccw
  arc A306 (-26.426, -20.9935) -> (-26.3475, -21.092) centre (0, 0) ccw
  arc A307 (-26.3244, -21.6857) -> (-26.3475, -21.092) centre (-26.7378, -21.4045) ccw
  arc A308 (-26.7993, -22.3307) -> (-26.3244, -21.6857) centre (-35.228, -15.6275) ccw
  arc A309 (-26.7993, -22.3307) -> (-26.8676, -22.4306) centre (-26.1505, -22.847) ccw
  arc A310 (-26.8676, -22.4306) -> (-27.3392, -23.331) centre (-16.7785, -28.2892) ccw
  arc A311 (-27.3392, -23.331) -> (-27.3246, -23.4386) centre (-27.2487, -23.3735) ccw
  arc A312 (-27.3246, -23.4386) -> (-26.8943, -23.931) centre (0, 0) ccw
  arc A313 (-26.8943, -23.931) -> (-26.7897, -23.96) centre (-26.8196, -23.8646) ccw
  arc A314 (-26.7897, -23.96) -> (-25.8342, -23.6135) centre (-30.2854, -12.8293) ccw
  arc A315 (-25.8342, -23.6135) -> (-25.726, -23.5592) centre (-26.1505, -22.847) ccw
  arc A316 (-25.0231, -23.1753) -> (-25.726, -23.5592) centre (-20.2148, -32.8115) ccw
  arc A317 (-24.4378, -23.2778) -> (-25.0231, -23.1753) centre (-24.7999, -23.6226) ccw
  arc A318 (-24.4378, -23.2778) -> (-24.3508, -23.3689) centre (0, 0) ccw
  arc A319 (-24.2746, -23.9582) -> (-24.3508, -23.3689) centre (-24.7115, -23.7151) ccw
  arc A320 (-24.6897, -24.6431) -> (-24.2746, -23.9582) centre (-33.6854, -18.7224) ccw
  arc A321 (-24.6897, -24.6431) -> (-24.7487, -24.7487) centre (-23.9973, -25.0992) ccw
  arc A322 (-24.7487, -24.7487) -> (-25.1378, -25.6877) centre (-14.1751, -29.6793) ccw
  arc A323 (-25.1378, -25.6877) -> (-25.1135, -25.7936) centre (-25.0438, -25.722) ccw
  arc A324 (-25.1135, -25.7936) -> (-24.6409, -26.2455) centre (0, 0) ccw
  arc A325 (-24.6409, -26.2455) -> (-24.5341, -26.2649) centre (-24.5725, -26.1726) ccw
  arc A326 (-24.5341, -26.2649) -> (-23.6135, -25.8342) centre (-29.0134, -15.4924) ccw
  arc A327 (-23.6135, -25.8342) -> (-23.5106, -25.7705) centre (-23.9973, -25.0992) ccw
  arc A328 (-22.845, -25.325) -> (-23.5106, -25.7705) centre (-17.1922, -34.4914) ccw
  arc A329 (-22.2528, -25.3747) -> (-22.845, -25.325) centre (-22.5825, -25.7506) ccw
  arc A330 (-22.2528, -25.3747) -> (-22.158, -25.4576) centre (0, 0) ccw
  arc A331 (-22.0293, -26.0377) -> (-22.158, -25.4576) centre (-22.4862, -25.8347) ccw
  arc A332 (-22.3813, -26.757) -> (-22.0293, -26.0377) centre (-31.8715, -21.6665) ccw
  arc A333 (-22.3813, -26.757) -> (-22.4306, -26.8676) centre (-21.6508, -27.1492) ccw
  arc A334 (-22.4306, -26.8676) -> (-22.7339, -27.8377) centre (-11.4577, -30.8305) ccw
  arc A335 (-22.7339, -27.8377) -> (-22.7003, -27.9409) centre (-22.6373, -27.8633) ccw
  arc A336 (-22.7003, -27.9409) -> (-22.1891, -28.3486) centre (0, 0) ccw
  arc A337 (-22.1891, -28.3486) -> (-22.0809, -28.3584) centre (-22.1275, -28.2699) ccw
  arc A338 (-22.0809, -28.3584) -> (-21.2027, -27.8469) centre (-27.5079, -18.0308) ccw
  arc A339 (-21.2027, -27.8469) -> (-21.1059, -27.7742) centre (-21.6508, -27.1492) ccw
  arc A340 (-20.4829, -27.2709) -> (-21.1059, -27.7742) centre (-14.0312, -35.8937) ccw
  arc A341 (-19.8887, -27.2672) -> (-20.4829, -27.2709) centre (-20.1833, -27.6712) ccw
  arc A342 (-19.8887, -27.2672) -> (-19.7868, -27.3413) centre (0, 0) ccw
  arc A343 (-19.6066, -27.9075) -> (-19.7868, -27.3413) centre (-20.0799, -27.7464) ccw
  arc A344 (-19.8928, -28.6556) -> (-19.6066, -27.9075) centre (-29.801, -24.4362) ccw
  arc A345 (-19.8928, -28.6556) -> (-19.932, -28.7701) centre (-19.13, -28.9807) ccw
  arc A346 (-19.932, -28.7701) -> (-20.1471, -29.7634) centre (-8.6479, -31.7334) ccw
  arc A347 (-20.1471, -29.7634) -> (-20.1043, -29.8633) centre (-20.0485, -29.7803) ccw
  arc A348 (-20.1043, -29.8633) -> (-19.5586, -30.2235) centre (0, 0) ccw
  arc A349 (-19.5586, -30.2235) -> (-19.45, -30.2236) centre (-19.5043, -30.1396) ccw
  arc A350 (-19.45, -30.2236) -> (-18.6211, -29.6353) centre (-25.7809, -20.424) ccw
  arc A351 (-18.6211, -29.6353) -> (-18.5312, -29.5543) centre (-19.13, -28.9807) ccw
  arc A352 (-17.9559, -28.9971) -> (-18.5312, -29.5543) centre (-10.7572, -37.0069) ccw
  arc A353 (-17.3644, -28.9403) -> (-17.9559, -28.9971) centre (-17.6216, -29.369) ccw
  arc A354 (-17.3644, -28.9403) -> (-17.2562, -29.0049) centre (0, 0) ccw
  arc A355 (-17.026, -29.5527) -> (-17.2562, -29.0049) centre (-17.5119, -29.4346) ccw
  arc A356 (-17.244, -30.3234) -> (-17.026, -29.5527) centre (-27.4906, -27.0092) ccw
  arc A357 (-17.244, -30.3234) -> (-17.2728, -30.4409) centre (-16.4552, -30.5788) ccw
  arc A358 (-17.2728, -30.4409) -> (-17.398, -31.4496) centre (-5.7685, -32.3808) ccw
  arc A359 (-17.398, -31.4496) -> (-17.3465, -31.5452) centre (-17.2983, -31.4576) ccw
  arc A360 (-17.3465, -31.5452) -> (-16.7707, -31.8551) centre (0, 0) ccw
  arc A361 (-16.7707, -31.8551) -> (-16.6625, -31.8454) centre (-16.7241, -31.7666) ccw
  arc A362 (-16.6625, -31.8454) -> (-15.8897, -31.1852) centre (-23.8463, -22.6528) ccw
  arc A363 (-15.8897, -31.1852) -> (-15.8074, -31.0964) centre (-16.4552, -30.5788) ccw
  arc A364 (-15.2843, -30.49) -> (-15.8074, -31.0964) centre (-7.3967, -37.8222) ccw
  arc A365 (-14.7003, -30.3803) -> (-15.2843, -30.49) centre (-14.9181, -30.8304) ccw
  arc A366 (-14.7003, -30.3803) -> (-14.5868, -30.435) centre (0, 0) ccw
  arc A367 (-14.3084, -30.9599) -> (-14.5868, -30.435) centre (-14.8029, -30.8859) ccw
  arc A368 (-14.4564, -31.747) -> (-14.3084, -30.9599) centre (-24.9588, -29.3647) ccw
  arc A369 (-14.4564, -31.747) -> (-14.4745, -31.8667) centre (-13.6479, -31.9307) ccw
  arc A370 (-14.4745, -31.8667) -> (-14.5088, -32.8825) centre (-2.8427, -32.7676) ccw
  arc A371 (-14.5088, -32.8825) -> (-14.449, -32.9731) centre (-14.4088, -32.8815) ccw
  arc A372 (-14.449, -32.9731) -> (-13.8477, -33.2301) centre (0, 0) ccw
  arc A373 (-13.8477, -33.2301) -> (-13.7408, -33.2108) centre (-13.8092, -33.1378) ccw
  arc A374 (-13.7408, -33.2108) -> (-13.0303, -32.484) centre (-21.7197, -24.6991) ccw
  arc A375 (-13.0303, -32.484) -> (-12.9563, -32.3882) centre (-13.6479, -31.9307) ccw
  arc A376 (-12.4897, -31.7373) -> (-12.9563, -32.3882) centre (-3.9765, -38.333) ccw
  arc A377 (-11.9179, -31.5757) -> (-12.4897, -31.7373) centre (-12.0944, -32.0435) ccw
  arc A378 (-11.9179, -31.5757) -> (-11.7999, -31.62) centre (0, 0) ccw
  arc A379 (-11.4756, -32.1179) -> (-11.7999, -31.62) centre (-11.9747, -32.0885) ccw
  arc A380 (-11.5524, -32.9151) -> (-11.4756, -32.1179) centre (-22.2261, -31.4838) ccw
  arc A381 (-11.5524, -32.9151) -> (-11.5598, -33.0359) centre (-10.7307, -33.0256) ccw
  arc A382 (-11.5598, -33.0359) -> (-11.5028, -34.0507) centre (0.106, -32.8905) ccw
  arc A383 (-11.5028, -34.0507) -> (-11.4351, -34.1356) centre (-11.4033, -34.0408) ccw
  arc A384 (-11.4351, -34.1356) -> (-10.8132, -34.3377) centre (0, 0) ccw
  arc A385 (-10.8132, -34.3377) -> (-10.7085, -34.3088) centre (-10.7832, -34.2423) ccw
  arc A386 (-10.7085, -34.3088) -> (-10.066, -33.5213) centre (-19.4183, -26.5467) ccw
  arc A387 (-10.066, -33.5213) -> (-10.0009, -33.4192) centre (-10.7307, -33.0256) ccw
  arc A388 (-9.5945, -32.7291) -> (-10.0009, -33.4192) centre (-0.5244, -38.5351) ccw
  arc A389 (-9.0395, -32.5169) -> (-9.5945, -32.7291) centre (-9.1734, -32.9987) ccw
  arc A390 (-9.0395, -32.5169) -> (-8.918, -32.5504) centre (0, 0) ccw
  arc A391 (-8.5504, -33.0173) -> (-8.918, -32.5504) centre (-9.0501, -33.0327) ccw
  arc A392 (-8.5554, -33.8182) -> (-8.5504, -33.0173) centre (-19.3145, -33.3494) ccw
  arc A393 (-8.5554, -33.8182) -> (-8.5519, -33.9391) centre (-7.7271, -33.8545) ccw
  arc A394 (-8.5519, -33.9391) -> (-8.4042, -34.9447) centre (3.0538, -32.7486) ccw
  arc A395 (-8.4042, -34.9447) -> (-8.3292, -35.0232) centre (-8.306, -34.9259) ccw
  arc A396 (-8.3292, -35.0232) -> (-7.6917, -35.1687) centre (0, 0) ccw
  arc A397 (-7.6917, -35.1687) -> (-7.59, -35.1306) centre (-7.6703, -35.071) ccw
  arc A398 (-7.59, -35.1306) -> (-7.0206, -34.2886) centre (-16.9605, -28.1804) ccw
  arc A399 (-7.0206, -34.2886) -> (-6.965, -34.1812) centre (-7.7271, -33.8545) ccw
  arc A400 (-6.622, -33.4574) -> (-6.965, -34.1812) centre (2.932, -38.427) ccw
  arc A401 (-6.0883, -33.1963) -> (-6.622, -33.4574) centre (-6.1785, -33.6881) ccw
  arc A402 (-6.0883, -33.1963) -> (-5.9643, -33.2188) centre (0, 0) ccw
  arc A403 (-5.5563, -33.6508) -> (-5.9643, -33.2188) centre (-6.0527, -33.7109) ccw
  arc A404 (-5.4896, -34.4489) -> (-5.5563, -33.6508) centre (-16.2473, -34.9465) ccw
  arc A405 (-5.4896, -34.4489) -> (-5.4752, -34.5691) centre (-4.6613, -34.4109) ccw
  arc A406 (-5.4752, -34.5691) -> (-5.238, -35.5574) centre (5.9771, -32.343) ccw
  arc A407 (-5.238, -35.5574) -> (-5.1562, -35.6288) centre (-5.1419, -35.5299) ccw
  arc A408 (-5.1562, -35.6288) -> (-4.5082, -35.7166) centre (0, 0) ccw
  arc A409 (-4.5082, -35.7166) -> (-4.4104, -35.6695) centre (-4.4957, -35.6174) ccw
  arc A410 (-4.4104, -35.6695) -> (-3.9188, -34.7799) centre (-14.3661, -29.5873) ccw
  arc A411 (-3.9188, -34.7799) -> (-3.8729, -34.6679) centre (-4.6613, -34.4109) ccw
  arc A412 (-3.5963, -33.9163) -> (-3.8729, -34.6679) centre (6.3647, -38.0095) ccw
  arc A413 (-3.0881, -33.6084) -> (-3.5963, -33.9163) centre (-3.1338, -34.1063) ccw
  arc A414 (-3.0881, -33.6084) -> (-2.9626, -33.6197) centre (0, 0) ccw
  arc A415 (-2.5175, -34.0134) -> (-2.9626, -33.6197) centre (-3.0065, -34.1178) ccw
  arc A416 (-2.3795, -34.8023) -> (-2.5175, -34.0134) centre (-13.0493, -36.2622) ccw
  arc A417 (-2.3795, -34.8023) -> (-2.3544, -34.9207) centre (-1.5579, -34.6902) ccw
  arc A418 (-2.3544, -34.9207) -> (-2.0296, -35.8838) centre (8.8523, -31.677) ccw
  arc A419 (-2.0296, -35.8838) -> (-1.9417, -35.9476) centre (-1.9363, -35.8477) ccw
  arc A420 (-1.9417, -35.9476) -> (-1.2884, -35.9769) centre (0, 0) ccw
  arc A421 (-1.2884, -35.9769) -> (-1.1952, -35.9213) centre (-1.2849, -35.877) ccw
  arc A422 (-1.1952, -35.9213) -> (-0.7853, -34.9912) centre (-11.6561, -30.756) ccw
  arc A423 (-0.7853, -34.9912) -> (-0.7497, -34.8755) centre (-1.5579, -34.6902) ccw
  arc A424 (-0.5416, -34.1021) -> (-0.7497, -34.8755) centre (9.7463, -37.2859) ccw
  arc A425 (-0.063, -33.7499) -> (-0.5416, -34.1021) centre (-0.0639, -34.2499) ccw
  arc A426 (-0.063, -33.7499) -> (0.063, -33.7499) centre (0, 0) ccw
  arc A427 (0.5416, -34.1021) -> (0.063, -33.7499) centre (0.0639, -34.2499) ccw
  arc A428 (0.7497, -34.8755) -> (0.5416, -34.1021) centre (-9.7463, -37.2859) ccw
  arc A429 (0.7497, -34.8755) -> (0.7853, -34.9912) centre (1.5579, -34.6902) ccw
  arc A430 (0.7853, -34.9912) -> (1.1952, -35.9213) centre (11.6561, -30.756) ccw
  arc A431 (1.1952, -35.9213) -> (1.2884, -35.9769) centre (1.2849, -35.877) ccw
  arc A432 (1.2884, -35.9769) -> (1.9417, -35.9476) centre (0, 0) ccw
  arc A433 (1.9417, -35.9476) -> (2.0296, -35.8838) centre (1.9363, -35.8477) ccw
  arc A434 (2.0296, -35.8838) -> (2.3544, -34.9207) centre (-8.8523, -31.677) ccw
  arc A435 (2.3544, -34.9207) -> (2.3795, -34.8023) centre (1.5579, -34.6902) ccw
  arc A436 (2.5175, -34.0134) -> (2.3795, -34.8023) centre (13.0493, -36.2622) ccw
  arc A437 (2.9626, -33.6197) -> (2.5175, -34.0134) centre (3.0065, -34.1178) ccw
  arc A438 (2.9626, -33.6197) -> (3.0881, -33.6084) centre (0, 0) ccw
  arc A439 (3.5963, -33.9163) -> (3.0881, -33.6084) centre (3.1338, -34.1063) ccw
  arc A440 (3.8729, -34.6679) -> (3.5963, -33.9163) centre (-6.3647, -38.0095) ccw
  arc A441 (3.8729, -34.6679) -> (3.9188, -34.7799) centre (4.6613, -34.4109) ccw
  arc A442 (3.9188, -34.7799) -> (4.4104, -35.6695) centre (14.3661, -29.5873) ccw
  arc A443 (4.4104, -35.6695) -> (4.5082, -35.7166) centre (4.4957, -35.6174) ccw
  arc A444 (4.5082, -35.7166) -> (5.1562, -35.6288) centre (0, 0) ccw
  arc A445 (5.1562, -35.6288) -> (5.238, -35.5574) centre (5.1419, -35.5299) ccw
  arc A446 (5.238, -35.5574) -> (5.4752, -34.5691) centre (-5.9771, -32.343) ccw
  arc A447 (5.4752, -34.5691) -> (5.4896, -34.4489) centre (4.6613, -34.4109) ccw
  arc A448 (5.5563, -33.6508) -> (5.4896, -34.4489) centre (16.2473, -34.9465) ccw
  arc A449 (5.9643, -33.2188) -> (5.5563, -33.6508) centre (6.0527, -33.7109) ccw
  arc A450 (5.9643, -33.2188) -> (6.0883, -33.1963) centre (0, 0) ccw
  arc A451 (6.622, -33.4574) -> (6.0883, -33.1963) centre (6.1785, -33.6881) ccw
  arc A452 (6.965, -34.1812) -> (6.622, -33.4574) centre (-2.932, -38.427) ccw
  arc A453 (6.965, -34.1812) -> (7.0206, -34.2886) centre (7.7271, -33.8545) ccw
  arc A454 (7.0206, -34.2886) -> (7.59, -35.1306) centre (16.9605, -28.1804) ccw
  arc A455 (7.59, -35.1306) -> (7.6917, -35.1687) centre (7.6703, -35.071) ccw
  arc A456 (7.6917, -35.1687) -> (8.3292, -35.0232) centre (0, 0) ccw
  arc A457 (8.3292, -35.0232) -> (8.4042, -34.9447) centre (8.306, -34.9259) ccw
  arc A458 (8.4042, -34.9447) -> (8.5519, -33.9391) centre (-3.0538, -32.7486) ccw
  arc A459 (8.5519, -33.9391) -> (8.5554, -33.8182) centre (7.7271, -33.8545) ccw
  arc A460 (8.5504, -33.0173) -> (8.5554, -33.8182) centre (19.3145, -33.3494) ccw
  arc A461 (8.918, -32.5504) -> (8.5504, -33.0173) centre (9.0501, -33.0327) ccw
  arc A462 (8.918, -32.5504) -> (9.0395, -32.5169) centre (0, 0) ccw
  arc A463 (9.5945, -32.7291) -> (9.0395, -32.5169) centre (9.1734, -32.9987) ccw
  arc A464 (10.0009, -33.4192) -> (9.5945, -32.7291) centre (0.5244, -38.5351) ccw
  arc A465 (10.0009, -33.4192) -> (10.066, -33.5213) centre (10.7307, -33.0256) ccw
  arc A466 (10.066, -33.5213) -> (10.7085, -34.3088) centre (19.4183, -26.5467) ccw
  arc A467 (10.7085, -34.3088) -> (10.8132, -34.3377) centre (10.7832, -34.2423) ccw
  arc A468 (10.8132, -34.3377) -> (11.4351, -34.1356) centre (0, 0) ccw
  arc A469 (11.4351, -34.1356) -> (11.5028, -34.0507) centre (11.4033, -34.0408) ccw
  arc A470 (11.5028, -34.0507) -> (11.5598, -33.0359) centre (-0.106, -32.8905) ccw
  arc A471 (11.5598, -33.0359) -> (11.5524, -32.9151) centre (10.7307, -33.0256) ccw
  arc A472 (11.4756, -32.1179) -> (11.5524, -32.9151) centre (22.2261, -31.4838) ccw
  arc A473 (11.7999, -31.62) -> (11.4756, -32.1179) centre (11.9747, -32.0885) ccw
  arc A474 (11.7999, -31.62) -> (11.9179, -31.5757) centre (0, 0) ccw
  arc A475 (12.4897, -31.7373) -> (11.9179, -31.5757) centre (12.0944, -32.0435) ccw
  arc A476 (12.9563, -32.3882) -> (12.4897, -31.7373) centre (3.9765, -38.333) ccw
  arc A477 (12.9563, -32.3882) -> (13.0303, -32.484) centre (13.6479, -31.9307) ccw
  arc A478 (13.0303, -32.484) -> (13.7408, -33.2108) centre (21.7197, -24.6991) ccw
  arc A479 (13.7408, -33.2108) -> (13.8477, -33.2301) centre (13.8092, -33.1378) ccw
  arc A480 (13.8477, -33.2301) -> (14.449, -32.9731) centre (0, 0) ccw
  arc A481 (14.449, -32.9731) -> (14.5088, -32.8825) centre (14.4088, -32.8815) ccw
  arc A482 (14.5088, -32.8825) -> (14.4745, -31.8667) centre (2.8427, -32.7676) ccw
  arc A483 (14.4745, -31.8667) -> (14.4564, -31.747) centre (13.6479, -31.9307) ccw
  arc A484 (14.3084, -30.9599) -> (14.4564, -31.747) centre (24.9588, -29.3647) ccw
  arc A485 (14.5868, -30.435) -> (14.3084, -30.9599) centre (14.8029, -30.8859) ccw
  arc A486 (14.5868, -30.435) -> (14.7003, -30.3803) centre (0, 0) ccw
  arc A487 (15.2843, -30.49) -> (14.7003, -30.3803) centre (14.9181, -30.8304) ccw
  arc A488 (15.8074, -31.0964) -> (15.2843, -30.49) centre (7.3967, -37.8222) ccw
  arc A489 (15.8074, -31.0964) -> (15.8897, -31.1852) centre (16.4552, -30.5788) ccw
  arc A490 (15.8897, -31.1852) -> (16.6625, -31.8454) centre (23.8463, -22.6528) ccw
  arc A491 (16.6625, -31.8454) -> (16.7707, -31.8551) centre (16.7241, -31.7666) ccw
  arc A492 (16.7707, -31.8551) -> (17.3465, -31.5452) centre (0, 0) ccw
  arc A493 (17.3465, -31.5452) -> (17.398, -31.4496) centre (17.2983, -31.4576) ccw
  arc A494 (17.398, -31.4496) -> (17.2728, -30.4409) centre (5.7685, -32.3808) ccw
  arc A495 (17.2728, -30.4409) -> (17.244, -30.3234) centre (16.4552, -30.5788) ccw
  arc A496 (17.026, -29.5527) -> (17.244, -30.3234) centre (27.4906, -27.0092) ccw
  arc A497 (17.2562, -29.0049) -> (17.026, -29.5527) centre (17.5119, -29.4346) ccw
  arc A498 (17.2562, -29.0049) -> (17.3644, -28.9403) centre (0, 0) ccw
  arc A499 (17.9559, -28.9971) -> (17.3644, -28.9403) centre (17.6216, -29.369) ccw
  arc A500 (18.5312, -29.5543) -> (17.9559, -28.9971) centre (10.7572, -37.0069) ccw
  arc A501 (18.5312, -29.5543) -> (18.6211, -29.6353) centre (19.13, -28.9807) ccw
  arc A502 (18.6211, -29.6353) -> (19.45, -30.2236) centre (25.7809, -20.424) ccw
  arc A503 (19.45, -30.2236) -> (19.5586, -30.2235) centre (19.5043, -30.1396) ccw
  arc A504 (19.5586, -30.2235) -> (20.1043, -29.8633) centre (0, 0) ccw
  arc A505 (20.1043, -29.8633) -> (20.1471, -29.7634) centre (20.0485, -29.7803) ccw
  arc A506 (20.1471, -29.7634) -> (19.932, -28.7701) centre (8.6479, -31.7334) ccw
  arc A507 (19.932, -28.7701) -> (19.8928, -28.6556) centre (19.13, -28.9807) ccw
  arc A508 (19.6066, -27.9075) -> (19.8928, -28.6556) centre (29.801, -24.4362) ccw
  arc A509 (19.7868, -27.3413) -> (19.6066, -27.9075) centre (20.0799, -27.7464) ccw
  arc A510 (19.7868, -27.3413) -> (19.8887, -27.2672) centre (0, 0) ccw
  arc A511 (20.4829, -27.2709) -> (19.8887, -27.2672) centre (20.1833, -27.6712) ccw
  arc A512 (21.1059, -27.7742) -> (20.4829, -27.2709) centre (14.0312, -35.8937) ccw
  arc A513 (21.1059, -27.7742) -> (21.2027, -27.8469) centre (21.6508, -27.1492) ccw
  arc A514 (21.2027, -27.8469) -> (22.0809, -28.3584) centre (27.5079, -18.0308) ccw
  arc A515 (22.0809, -28.3584) -> (22.1891, -28.3486) centre (22.1275, -28.2699) ccw
  arc A516 (22.1891, -28.3486) -> (22.7003, -27.9409) centre (0, 0) ccw
  arc A517 (22.7003, -27.9409) -> (22.7339, -27.8377) centre (22.6373, -27.8633) ccw
  arc A518 (22.7339, -27.8377) -> (22.4306, -26.8676) centre (11.4577, -30.8305) ccw
  arc A519 (22.4306, -26.8676) -> (22.3813, -26.757) centre (21.6508, -27.1492) ccw
  arc A520 (22.0293, -26.0377) -> (22.3813, -26.757) centre (31.8715, -21.6665) ccw
  arc A521 (22.158, -25.4576) -> (22.0293, -26.0377) centre (22.4862, -25.8347) ccw
  arc A522 (22.158, -25.4576) -> (22.2528, -25.3747) centre (0, 0) ccw
  arc A523 (22.845, -25.325) -> (22.2528, -25.3747) centre (22.5825, -25.7506) ccw
  arc A524 (23.5106, -25.7705) -> (22.845, -25.325) centre (17.1922, -34.4914) ccw
  arc A525 (23.5106, -25.7705) -> (23.6135, -25.8342) centre (23.9973, -25.0992) ccw
  arc A526 (23.6135, -25.8342) -> (24.5341, -26.2649) centre (29.0134, -15.4924) ccw
  arc A527 (24.5341, -26.2649) -> (24.6409, -26.2455) centre (24.5725, -26.1726) ccw
  arc A528 (24.6409, -26.2455) -> (25.1135, -25.7936) centre (0, 0) ccw
  arc A529 (25.1135, -25.7936) -> (25.1378, -25.6877) centre (25.0438, -25.722) ccw
  arc A530 (25.1378, -25.6877) -> (24.7487, -24.7487) centre (14.1751, -29.6793) ccw
  arc A531 (24.7487, -24.7487) -> (24.6897, -24.6431) centre (23.9973, -25.0992) ccw
  arc A532 (24.2746, -23.9582) -> (24.6897, -24.6431) centre (33.6854, -18.7224) ccw
  arc A533 (24.3508, -23.3689) -> (24.2746, -23.9582) centre (24.7115, -23.7151) ccw
  arc A534 (24.3508, -23.3689) -> (24.4378, -23.2778) centre (0, 0) ccw
  arc A535 (25.0231, -23.1753) -> (24.4378, -23.2778) centre (24.7999, -23.6226) ccw
  arc A536 (25.726, -23.5592) -> (25.0231, -23.1753) centre (20.2148, -32.8115) ccw
  arc A537 (25.726, -23.5592) -> (25.8342, -23.6135) centre (26.1505, -22.847) ccw
  arc A538 (25.8342, -23.6135) -> (26.7897, -23.96) centre (30.2854, -12.8293) ccw
  arc A539 (26.7897, -23.96) -> (26.8943, -23.931) centre (26.8196, -23.8646) ccw
  arc A540 (26.8943, -23.931) -> (27.3246, -23.4386) centre (0, 0) ccw
  arc A541 (27.3246, -23.4386) -> (27.3392, -23.331) centre (27.2487, -23.3735) ccw
  arc A542 (27.3392, -23.331) -> (26.8676, -22.4306) centre (16.7785, -28.2892) ccw
  arc A543 (26.8676, -22.4306) -> (26.7993, -22.3307) centre (26.1505, -22.847) ccw
  arc A544 (26.3244, -21.6857) -> (26.7993, -22.3307) centre (35.228, -15.6275) ccw
  arc A545 (26.3475, -21.092) -> (26.3244, -21.6857) centre (26.7378, -21.4045) ccw
  arc A546 (26.3475, -21.092) -> (26.426, -20.9935) centre (0, 0) ccw
  arc A547 (26.9998, -20.8389) -> (26.426, -20.9935) centre (26.8175, -21.3045) ccw
  arc A548 (27.7342, -21.1584) -> (26.9998, -20.8389) centre (23.0746, -30.8673) ccw
  arc A549 (27.7342, -21.1584) -> (27.8469, -21.2027) centre (28.0932, -20.4109) ccw
  arc A550 (27.8469, -21.2027) -> (28.8296, -21.4621) centre (31.3135, -10.0629) ccw
  arc A551 (28.8296, -21.4621) -> (28.9312, -21.4239) centre (28.8509, -21.3644) ccw
  arc A552 (28.9312, -21.4239) -> (29.3156, -20.8949) centre (0, 0) ccw
  arc A553 (29.3156, -20.8949) -> (29.3205, -20.7864) centre (29.2342, -20.8368) ccw
  arc A554 (29.3205, -20.7864) -> (28.7701, -19.932) centre (19.2468, -26.6713) ccw
  arc A555 (28.7701, -19.932) -> (28.6931, -19.8385) centre (28.0932, -20.4109) ccw
  arc A556 (28.1624, -19.2387) -> (28.6931, -19.8385) centre (36.487, -12.4067) ccw
  arc A557 (28.1321, -18.6453) -> (28.1624, -19.2387) centre (28.5489, -18.9215) ccw
  arc A558 (28.1321, -18.6453) -> (28.2015, -18.5402) centre (0, 0) ccw
  arc A559 (28.7591, -18.3348) -> (28.2015, -18.5402) centre (28.6193, -18.8148) ccw
  arc A560 (29.5192, -18.5871) -> (28.7591, -18.3348) centre (25.7486, -28.6747) ccw
  arc A561 (29.5192, -18.5871) -> (29.6353, -18.6211) centre (29.8098, -17.8105) ccw
  arc A562 (29.6353, -18.6211) -> (30.6374, -18.7914) centre (32.0894, -7.2155) ccw
  arc A563 (30.6374, -18.7914) -> (30.7352, -18.7443) centre (30.6498, -18.6922) ccw
  arc A564 (30.7352, -18.7443) -> (31.0706, -18.1829) centre (0, 0) ccw